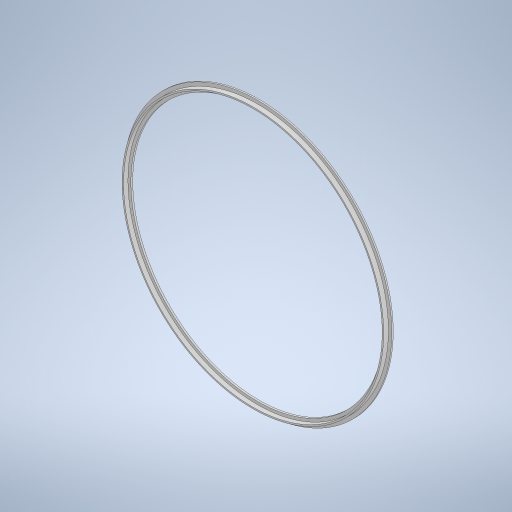
# Autodesk Inventor part: Spacer
Saved by Autodesk Inventor 2024 (Build 280153000, 153)
## iProperties
Created: 2024-01-24
Part Number: Spacer
Material: Generic
Document SubType Name: Modeling
Designer: crow
Density: 1 g/cm^3
Appearance: Default
Mass: 111.898 g
Surface Area: 571.389 cm^2
Volume: 111.898 cm^3
Author: crow
## iProperties of the stored document Spacer_3DPrint.ipt
Created: 2024-01-24
Part Number: Spacer_3DPrint
Material: Generic
Document SubType Name: Modeling
Designer: crow
Density: 1 g/cm^3
Appearance: Default
Author: crow
Autodesk Inventor part; units mm, degrees
ref_plane "YZ Plane" through (0, 0, 0) normal (1, 0, 0) x (0, 1, 0)
ref_plane "XZ Plane" through (0, 0, 0) normal (0, 1, 0) x (-1, 0, 0)
ref_plane "XY Plane" through (0, 0, 0) normal (0, 0, 1) x (1, 0, 0)
sketch "Sketch2" plane through (0, 0, 0) normal (1, 0, 0) x (0, 1, 0)
  line L0 (-93.3, 0) -> (-93.3, 1)
  line L1 (-93.3, 1) -> (-93.3, 0) projected
  line L2 (-93.3, 1) -> (-91, 1)
  line L3 (-91, 4.25) -> (-91, 1)
  line L4 (-91, 1) -> (-91, 4.25)
  line L5 (-91, 4.25) -> (-90, 4.25)
  line L6 (-90, 4.25) -> (-90, 1.25)
  line L7 (-90, 4.25) -> (-90, 1.25)
  line L8 (-90, 1.25) -> (-88, 1.25)
  line L9 (-88, 1.25) -> (-88, 0) projected
  line L10 (-88, 1.25) -> (-88, 0)
  line L11 (-1.5, 0) -> (-1.5, 31.2908) construction
  line L12 (-93.3, 0) -> (-88, 0)
  dimension "d0" = 1
  dimension "d2" = 3
  dimension "d3" = 2
  dimension "d4" = 3.25
  dimension "d5" = 1
  dimension "d7" = 91.8
  constraints: 22 end point, 5 point on line, 3 perpendicular, 2 vertical, 1 horizontal
  measures "d0" distance of L0.start L0.end
  measures "d2" distance of L6.start L6.end
  measures "d3" distance of L7.end L8.end
  measures "d4" distance of L3.start L3.end
  measures "d5" distance of L3.start L5.end
  measures "d7" distance between parallel lines of L11 L0
revolve "Revolution1" add sketch "Sketch2" angle 360 about axis through (0, -1.5, 0) along (0, 0, 1)
body "Solid3"
